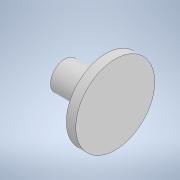
# Autodesk Inventor part: WheelInfillProfileV1
Saved by Autodesk Inventor 2020 (Build 240168000, 168)
## iProperties
Created: 2023-12-21
Part Number: WheelInfillProfileV1
Material: Generic
Document SubType Name: Modeling
Designer: smz3rm
Density: 1 g/cm^3
Appearance: Default
Author: smz3rm
Autodesk Inventor part; units mm, degrees
ref_plane "YZ Plane" through (0, 0, 0) normal (1, 0, 0) x (0, 1, 0)
ref_plane "XZ Plane" through (0, 0, 0) normal (0, 1, 0) x (-1, 0, 0)
ref_plane "XY Plane" through (0, 0, 0) normal (0, 0, 1) x (1, 0, 0)
sketch "Sketch1" plane through (0, 0, 0) normal (1, 0, 0) x (0, 1, 0)
  circle A0 centre (0, 0) radius 12.5
  dimension "d0" = 25
  constraints: 1 centre point, 1 coincident
  measures "d0" diameter of A0
extrude "Extrusion1" add sketch "Sketch1" along normal blind 3
sketch "Sketch2" plane through (0, 0, 0) normal (-1, 0, 0) x (0, 0, 1)
  circle A0 centre (0, 0) radius 4.5
  dimension "d3" = 9
  constraints: 1 centre point, 1 coincident
  measures "d3" diameter of A0
extrude "Extrusion2" add sketch "Sketch2" along normal blind 13
equation "\"d0\" = WheelGrooveDia"
equation "\"d1\" = WheelGrooveWidth"
equation "\"d4\" = WheelWidth"
equation "\"WheelGrooveDia\" = 25"
equation "\"WheelGrooveWidth\" = 3"
equation "\"WheelWidth\" = 13"
body "Solid1"
